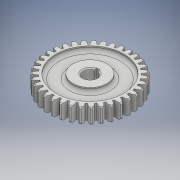
# Autodesk Inventor part: 도면2-4번
Saved by Autodesk Inventor 2018.3 (Build 223284000, 284)
## iProperties
Created: 2019-10-11
Part Number: 도면2-4번
Material: 일반
Document SubType Name: Modeling
Designer: MyTool
Density: 1 g/cm^3
Appearance: 기본값
Author: MyTool
Autodesk Inventor part; units mm, degrees
ref_plane "YZ Plane" through (0, 0, 0) normal (1, 0, 0) x (0, 1, 0)
ref_plane "XZ Plane" through (0, 0, 0) normal (0, 1, 0) x (-1, 0, 0)
ref_plane "XY Plane" through (0, 0, 0) normal (0, 0, 1) x (1, 0, 0)
sketch "스케치1" plane through (0, 0, 0) normal (0, 0, 1) x (1, 0, 0)
  circle A0 centre (0, 0) radius 35 construction
  circle A1 centre (0, 0) radius 37 construction
  circle A2 centre (0, 0) radius 32 construction
  line L0 (0, 37) -> (0, 0) construction
  line L1 (0.57, 36.9956) -> (0.57, 0) construction
  line L2 (1.57, 34.9648) -> (1.57, 0) construction
  line L3 (2.07, 31.933) -> (2.07, 0) construction
  arc A3 (2.07, 31.933) -> (0.57, 36.9956) centre (-7.0372, 31.9882) ccw
  arc A4 (-0.57, 36.9956) -> (-2.07, 31.933) centre (7.0372, 31.9882) ccw
  arc A5 (-2.07, 31.933) -> (2.07, 31.933) centre (0, 0) ccw
  arc A6 (0.57, 36.9956) -> (-0.57, 36.9956) centre (0, 0) ccw
  dimension "d0" = 70
  dimension "d2" = 64
  dimension "d1" = 74
  dimension "d3" = 1
  dimension "d4" = 0.5
  dimension "d5" = 1.57
  constraints: 11 point on circle, 8 end point, 5 centre point, 5 coincident, 4 vertical, 3 symmetric about line, 7 other
  measures "d1" diameter of A1
  measures "d3" distance between parallel lines of L2 L1
  measures "d4" distance between parallel lines of L3 L2
  measures "d5" distance between parallel lines of L0 L2
extrude "돌출1" add sketch "스케치1" along normal mid plane 13
chamfer "모따기1" distance 1 angle 45 2 edges at (0, 37, 6.5) (0, 37, -6.5)
pattern_circular "원형 패턴1" count 35 over 360 about axis through (0, 0, 0) along (0, 0, 1) of "돌출1", "모따기1"
sketch "스케치3" plane through (0, 0, -6.5) normal (0, 0, -1) x (-1, 0, 0)
  circle A0 centre (0, 0) radius 10
  dimension "d11" = 20
  constraints: 1 centre point, 1 coincident
  measures "d11" diameter of A0
extrude "돌출2" add sketch "스케치3" along normal blind 12
sketch "스케치4" plane through (0, 0, -18.5) normal (0, 0, -1) x (-1, 0, 0)
  circle A0 centre (0, 0) radius 6
  line L0 (-1.5, 0) -> (1.5, 0)
  line L1 (1.5, 0) -> (1.5, 7.4)
  line L2 (1.5, 7.4) -> (-1.5, 7.4)
  line L3 (-1.5, 7.4) -> (-1.5, 0)
  dimension "d14" = 12
  dimension "d15" = 1.5
  dimension "d16" = 3
  dimension "d17" = 1.4
  constraints: 8 end point, 2 parallel, 1 centre point, 1 coincident, 1 horizontal, 1 perpendicular
  measures "d14" diameter of A0
  measures "d15" distance from line of point (0, 0) L3
  measures "d16" distance of L0.start L0.end
  measures "d17" distance edge to line of A0 L2
extrude "돌출3" cut sketch "스케치4" against normal up to next
chamfer "모따기2" distance 1 angle 45 2 edges at (0, -6, -18.5) (0, -6, 6.5)
sketch "스케치5" plane through (0, 0, -6.5) normal (0, 0, -1) x (-1, 0, 0)
  circle A0 centre (0, 0) radius 15
  circle A1 centre (0, 0) radius 30
  dimension "d26" = 30
  dimension "d27" = 60
  constraints: 2 centre point, 2 coincident
  measures "d26" diameter of A0
  measures "d27" diameter of A1
extrude "돌출4" cut sketch "스케치5" against normal blind 4
mirror "미러1" about plane through (0, 0, 0) normal (0, 0, 1) of "돌출4"
fillet "모깎기1" radius 3 5 edges at (30, 0, -2.5) (15, 0, -2.5) (10, 0, -6.5) (30, 0, 2.5) (15, 0, 2.5)
sketch "스케치6" plane through (0, 0, 0) normal (0, 1, 0) x (-1, 0, 0)
  circle A0 centre (0, -15.5) radius 1.5
  line L0 (-7, -18.5) -> (7, -18.5) projected
  point P0 (0, 0)
  point P1 (-1.5, -18.5)
  point P2 (1.5, -18.5)
  dimension "d31" = 3
  dimension "d32" = 3
  constraints: 1 centre point
  measures "d31" diameter of A0
  measures "d32" distance from line of L0 A0.centre
hole "구멍1" at (0, 0, -15.5) direction (0, -1, 0) diameter 2.459 end through all thread size "M3x0.5" class "6H" standard "ANSI Metric M Profile"
equation "\"d15\" = 0.5 * d16"
